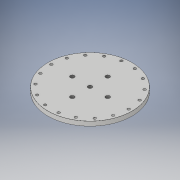
# Autodesk Inventor part: Deckelplatte
Saved by Autodesk Inventor 2017 (Build 210142000, 142)
## iProperties
Part Number: Deckelplatte
Material: Generisch
Document SubType Name: Modeling
Designer: Benjamin
Density: 1 g/cm^3
Appearance: Vorgabe
Author: Benjamin
Autodesk Inventor part; units mm, degrees
ref_plane "YZ Plane" through (0, 0, 0) normal (1, 0, 0) x (0, 1, 0)
ref_plane "XZ Plane" through (0, 0, 0) normal (0, 1, 0) x (-1, 0, 0)
ref_plane "XY Plane" through (0, 0, 0) normal (0, 0, 1) x (1, 0, 0)
sketch "Skizze1" plane through (0, 0, 0) normal (0, 0, 1) x (1, 0, 0)
  circle A0 centre (0, 0) radius 190
  dimension "d0" = 380
  constraints: 1 centre point, 1 coincident
  measures "d0" diameter of A0
extrude "Extrusion1" add sketch "Skizze1" along normal blind 20
sketch "Skizze2" plane through (0, 0, 0) normal (0, 0, -1) x (-1, 0, 0)
  circle A0 centre (0, 0) radius 144
  dimension "d3" = 288
  constraints: 1 centre point, 1 coincident
  measures "d3" diameter of A0
extrude "Extrusion2" add sketch "Skizze2" along normal blind 5
sketch "Skizze3" plane through (0, 0, 20) normal (0, 0, 1) x (1, 0, 0)
  point P0 (0, 0)
  point P1 (0, 0)
  point P2 (175, 0)
  constraints: 1 coincident
hole "Bohrung1" at (175, 0, 20) direction (0, 0, -1) diameter 11 depth 25 tip angle 118
pattern_circular "Runde Anordnung1" count 18 over 360 about axis through (0, 0, 0) along (0, 0, 1) of "Bohrung1"
sketch "Skizze4" plane through (0, 0, 20) normal (0, 0, 1) x (1, 0, 0)
  point P0 (0, 0)
  point P1 (0, 0)
  constraints: 1 coincident
hole "Bohrung2" at (0, 0, 20) direction (0, 0, -1) diameter 17.294 depth 51.2 tip angle 118 thread size "M20x2.5" class "6H" standard "ISO Metric profile"
sketch "Skizze5" plane through (0, 0, 20) normal (0, 0, 1) x (1, 0, 0)
  point P0 (0, 0)
  point P1 (80, 0)
hole "Bohrung3" at (80, 0, 20) direction (0, 0, -1) diameter 17.294 depth 51.2 tip angle 118 thread size "M20x2.5" class "6H" standard "ISO Metric profile"
pattern_circular "Runde Anordnung2" count 4 over 360 about axis through (0, 0, 0) along (0, 0, 1) of "Bohrung3"
chamfer "Fase1" distance 0.3 angle 45 48 edges at (144, 0, -5) (-190, 0, 0) (-24.972, -173.2964, 0) (35.8049, -171.3863, 0) (92.2631, -148.8044, 0) (137.5931, -108.2746, 0) (-82.7369, -154.3044, 0) (-130.5224, -116.7011, 0) (-162.5651, -65.0218, 0) (-175, -5.5, 0) (-166.3273, 54.6852, 0) (-137.5931, 108.2746, 0) (-92.2631, 148.8044, 0) (-35.8049, 171.3863, 0) (24.972, 173.2964, 0) (82.7369, 154.3044, 0) (162.5651, 65.0218, 0) (130.5224, 116.7011, 0) (175, 5.5, 0) (166.3273, -54.6852, 0) (80, 8.647, -5) (8.647, -80, -5) (-80, -8.647, -5) (-8.647, 80, -5) (0, 8.647, -5) (-175, -5.5, 20) (-166.3273, 54.6852, 20) (-137.5931, 108.2746, 20) (-92.2631, 148.8044, 20) (-35.8049, 171.3863, 20) (24.972, 173.2964, 20) (82.7369, 154.3044, 20) (130.5224, 116.7011, 20) (162.5651, 65.0218, 20) (175, 5.5, 20) (-162.5651, -65.0218, 20) (-130.5224, -116.7011, 20) (-82.7369, -154.3044, 20) (-24.972, -173.2964, 20) (35.8049, -171.3863, 20) (166.3273, -54.6852, 20) (137.5931, -108.2746, 20) (0, 8.647, 20) (92.2631, -148.8044, 20) (-80, -8.647, 20) (8.647, -80, 20) (80, 8.647, 20) (-8.647, 80, 20)
chamfer "Fase2" distance 0.3 angle 45 1 edges at (-190, 0, 20)
